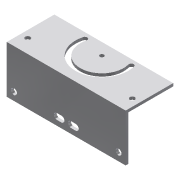
# Autodesk Inventor part: L profil
Saved by Autodesk Inventor 2015 (Build 190159000, 159)
## iProperties
Created: 2015-01-07
Part Number: L profil
Material: Všeobecné
Document SubType Name: Modeling
Designer: Michal
Density: 1 g/cm^3
Appearance: Hliník – leštěný
Author: Michal
Autodesk Inventor part; units mm, degrees
ref_plane "YZ Plane" through (0, 0, 0) normal (1, 0, 0) x (0, 1, 0)
ref_plane "XZ Plane" through (0, 0, 0) normal (0, 1, 0) x (-1, 0, 0)
ref_plane "XY Plane" through (0, 0, 0) normal (0, 0, 1) x (1, 0, 0)
sketch "Náčrt1" plane through (0, 0, 0) normal (1, 0, 0) x (0, 1, 0)
  line L0 (0, 0) -> (100, 0)
  line L1 (100, 0) -> (100, -6)
  line L2 (100, -6) -> (6, -6)
  line L3 (6, -6) -> (6, -100)
  line L4 (6, -100) -> (0, -100)
  line L5 (0, -100) -> (0, 0)
  point P0 (100, -148)
  point P1 (100, -150)
  dimension "d0" = 100
  dimension "d1" = 6
  dimension "d20" = 100
  dimension "d40" = 6
  dimension "d108" = 94
  dimension "d109" = 94
  constraints: 12 end point, 3 perpendicular, 2 point on line, 1 horizontal
  measures "d0" distance of L0.start L0.end
  measures "d1" distance of L0.end L1.end
  measures "d20" distance of L4.end L0.start
  measures "d40" distance of L3.end L4.end
  measures "d108" distance of L1.end L2.end
  measures "d109" distance of L2.end L3.end
extrude "Vysunutí1" add sketch "Náčrt1" along normal blind 140
sketch "Náčrt7" plane through (0, 6, -6) normal (0, 0, -1) x (-1, 0, 0)
  circle A0 centre (-125, 23) radius 5.25
  line L0 (0, 0) -> (-140, 0) projected
  line L1 (-140, 0) -> (-140, 94) projected
  line L2 (0, 94) -> (0, 0) projected
  point P0 (0, -6)
  dimension "d43" = 10.5
  dimension "d44" = 23
  dimension "d101" = 15
  constraints: 1 centre point
  measures "d43" diameter of A0
  measures "d44" distance from line of A0.centre L0
  measures "d101" distance from line of L1 A0.centre
extrude "Vysunutí6" cut sketch "Náčrt7" against normal through all
sketch "Náčrt11" plane through (0, 0, 0) normal (-1, 0, 0) x (0, 0, 1)
  line L0 (0, 0) -> (0, 100) projected
  line L1 (0, 100) -> (-6, 100) projected
  line L2 (-6, 100) -> (-6, 6) projected
  line L3 (-6, 6) -> (-100, 6) projected
  line L4 (-100, 6) -> (-100, 0) projected
  line L5 (-100, 0) -> (0, 0) projected
extrude "Vysunutí9" add sketch "Náčrt11" along normal blind 110
sketch "Náčrt9" plane through (0, 6, -6) normal (0, 1, 0) x (1, 0, 0)
  line L0 (140, 94) -> (-110, 94) projected
  line L1 (140, -6) -> (140, 94) projected
  line L2 (-110, -6) -> (140, -6) projected
  line L3 (0, -6) -> (140, -6) projected
  arc A0 (5, 70.75) -> (5, 83.25) centre (5, 77) ccw
  arc A1 (-5, 83.25) -> (-5, 70.75) centre (-5, 77) ccw
  line L4 (-5, 70.75) -> (5, 70.75)
  line L5 (5, 83.25) -> (-5, 83.25)
  line L6 (-110, 94) -> (-110, -6) projected
  point P0 (0, -3)
  point P1 (0, 77)
  dimension "d89" = 140
  dimension "d91" = 12.5
  dimension "d92" = 12.5
  dimension "d93" = 10
  dimension "d94" = 5
  dimension "d106" = 17
  constraints: 4 end point, 4 point on circle, 2 centre point, 1 parallel, 1 tangent, 1 other
  measures "d89" distance from line of L1 point (0, 77)
  measures "d91" diameter of A0
  measures "d92" diameter of A1
  measures "d93" distance of A1.centre A0.centre
  measures "d94" distance of point (0, 77) A0.centre
  measures "d106" distance from line of L0 point (0, 77)
sketch "Náčrt10" plane through (0, 0, 0) normal (0, 0, 1) x (1, 0, 0)
  line L0 (0, 100) -> (140, 100) projected
  circle A0 centre (125, 29) radius 5.25 projected
  circle A1 centre (15, 75) radius 4.25
  arc A2 (-28.9496, 86.7763) -> (58.9496, 86.7763) centre (15, 75) ccw
  arc A3 (-38.6089, 89.3645) -> (68.6089, 89.3645) centre (15, 75) ccw
  arc A4 (68.6089, 89.3645) -> (58.9496, 86.7763) centre (63.7793, 88.0704) ccw
  line L1 (15, 75) -> (84.9162, 75)
  line L2 (15, 75) -> (59.3726, 86.8896)
  line L3 (15, 75) -> (15, -2.5844)
  line L4 (15, 75) -> (-28.9496, 86.7763)
  arc A5 (-28.9496, 86.7763) -> (-38.6089, 89.3645) centre (-33.7793, 88.0704) ccw
  line L5 (140, 100) -> (140, 0) projected
  line L6 (0, 0) -> (140, 0) projected
  dimension "d66" = 8.5
  dimension "d67" = 91
  dimension "d68" = 111
  dimension "d69" = 10
  dimension "d70" = 10
  dimension "d73" = 15
  dimension "d74" = 105
  dimension "d78" = 10
  dimension "d83" = 125
  dimension "d84" = 75
  constraints: 8 end point, 8 point on circle, 5 centre point, 2 coincident, 2 tangent, 1 horizontal, 1 point on line, 1 vertical
  measures "d66" diameter of A1
  measures "d67" diameter of A2
  measures "d68" diameter of A3
  measures "d69" radial gap between concentric circles of A3 A2
  measures "d70" diameter of A4
  measures "d73" angle of L1 L2
  measures "d74" angle of L3 L4
  measures "d78" diameter of A5
  measures "d83" distance from line of L5 A1.centre
  measures "d84" distance from line of L6 A1.centre
extrude "Vysunutí13" cut sketch "Náčrt9" against normal through all contours L4 A1 L5 A0
extrude "Vysunutí14" cut sketch "Náčrt10" against normal through all contours L1 L2 A1 | A1 L3 L1 | L2 L4 A1 | A1 L4 L3 | L1 A3 L3 A2 | A2 A4 A3 L1 | L3 A3 A5 A2
ref_plane "Pracovní rovina2" through (15, 0, 0) normal (1, 0, 0) x (0, 0, -1)
mirror "Zrcadlit2" about plane through (15, 0, 0) normal (1, 0, 0) of "Vysunutí13", "Vysunutí6"
sketch "Náčrt12" plane through (140, 6, -6) normal (0, 1, 0) x (1, 0, 0)
  line L0 (-115, 83.25) -> (-105, 83.25) projected
  arc A0 (-105, 70.75) -> (-105, 83.25) centre (-105, 77) ccw projected
  line L1 (-105, 70.75) -> (-115, 70.75) projected
  arc A1 (-115, 83.25) -> (-115, 70.75) centre (-115, 77) ccw projected
  line L2 (-135, 70.75) -> (-145, 70.75) projected
  arc A2 (-145, 83.25) -> (-145, 70.75) centre (-145, 77) ccw projected
  line L3 (-145, 83.25) -> (-135, 83.25) projected
  arc A3 (-135, 70.75) -> (-135, 83.25) centre (-135, 77) ccw projected
  line L4 (0, 0) -> (-250, 0) projected
  line L5 (0, 94) -> (0, 0) projected
  line L6 (0, 94) -> (-250, 94) projected
  line L7 (-250, 0) -> (-250, 94) projected
  circle A4 centre (-15, 77) radius 6.25
  point P0 (-140, -6)
  dimension "d102" = 12.5
  dimension "d103" = 15
  dimension "d107" = 17
  constraints: 1 centre point
  measures "d102" diameter of A4
  measures "d103" distance from line of L5 A4.centre
  measures "d107" distance from line of L6 A4.centre
extrude "Vysunutí15" cut sketch "Náčrt12" against normal through all contours A4
mirror "Zrcadlit3" about plane through (15, 0, 0) normal (1, 0, 0) of "Vysunutí15"
